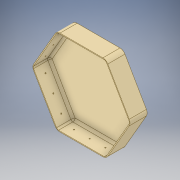
# Autodesk Inventor part: Base
Saved by Autodesk Inventor 2019 (Build 230136000, 136)
## iProperties
Created: 2021-07-14
Part Number: Base
Material: Generic
Document SubType Name: Modeling
Designer: Lix
Density: 1 g/cm^3
Appearance: Beige
Author: Lix
Autodesk Inventor part; units mm, degrees
ref_plane "YZ Plane" through (0, 0, 0) normal (1, 0, 0) x (0, 1, 0)
ref_plane "XZ Plane" through (0, 0, 0) normal (0, 1, 0) x (-1, 0, 0)
ref_plane "XY Plane" through (0, 0, 0) normal (0, 0, 1) x (1, 0, 0)
sketch "Sketch1" plane through (0, 0, 0) normal (0, 0, 1) x (1, 0, 0)
  line L0 (43.3013, -75) -> (-43.3013, -75)
  line L1 (-43.3013, -75) -> (-86.6025, 0)
  line L2 (-86.6025, 0) -> (-43.3013, 75)
  line L3 (-43.3013, 75) -> (43.3013, 75)
  line L4 (43.3013, 75) -> (86.6025, 0)
  line L5 (86.6025, 0) -> (43.3013, -75)
  point P0 (0, 0)
  point P1 (0, 0)
  dimension "d0" = 150
  constraints: 12 end point, 1 coincident, 1 horizontal, 13 other
  measures "d0" distance between parallel lines of L5 L2
extrude "Extrusion1" add sketch "Sketch1" along normal blind 30
shell "Shell1" thickness 1.5 removed faces 1 at (14.4338, -25, 30) ; own thickness 1 on faces at (14.4338, -25, 0)
sketch "Sketch2" plane through (-84.8705, 0, 30) normal (0.8660254, 0.5, 0) x (0, 0, -1)
  circle A0 centre (14.5, -69.8705) radius 1
  circle A1 centre (14.5, -15) radius 1
  line L0 (29, -84.8705) -> (0, -84.8705) projected
  line L1 (29, 0) -> (0, 0) projected
  circle A2 centre (14.5, -42.4352) radius 1
  line L2 (29, -84.8705) -> (29, 0) projected
  line L3 (29, 0) -> (0, 0) projected
  line L4 (0, -84.8705) -> (0, 0) projected
  line L5 (29, -84.8705) -> (0, -84.8705) projected
  line L6 (0, -84.8705) -> (0, 0) projected
  point P0 (30, -42.4352)
  point P1 (14.5, -84.8705)
  point P2 (0, -42.4352)
  dimension "d5" = 2
  dimension "d6" = 15
  dimension "d7" = 15
  constraints: 3 centre point, 3 vertical alignment, 2 equal radius, 2 midpoint, 1 horizontal alignment
  measures "d5" diameter of A0
  measures "d6" distance of A0.centre point (14.5, -84.87)
  measures "d7" distance from line of L1 A1.centre
ref_plane "Work Plane1" through (-21.6506, 37.5, 30) normal (0.8660254, 0.5, 0) x (0, 0, -1)
ref_plane "Work Plane2" through (-43.3013, 0, 0) normal (0, 1, 0) x (1, 0, 0)
ref_plane "Work Plane3" through (-21.6506, -37.5, 0) normal (-0.8660254, 0.5, 0) x (0, 0, 1)
extrude "Extrusion2" cut sketch "Sketch2" against normal blind 1 contours A0 | A1 | A2
mirror "Mirror1" about plane through (-21.6506, 37.5, 30) normal (0.8660254, 0.5, 0) of "Extrusion2"
mirror "Mirror2" about plane through (-43.3013, 0, 0) normal (0, 1, 0) of "Extrusion2"
mirror "Mirror3" about plane through (-21.6506, -37.5, 0) normal (-0.8660254, 0.5, 0) of "Extrusion2", "Mirror2"
mirror "Mirror4" about plane through (-43.3013, 0, 0) normal (0, 1, 0) of "Extrusion2", "Mirror2", "Mirror3"
fillet "Fillet1" radius 4 12 edges at (0, -73.5, 1) (-63.6529, -36.75, 1) (63.6529, -36.75, 1) (63.6529, 36.75, 1) (0, 73.5, 1) (-63.6529, 36.75, 1) (-84.8705, 0, 15.5) (-42.4352, 73.5, 15.5) (42.4352, 73.5, 15.5) (84.8705, 0, 15.5) (42.4352, -73.5, 15.5) (-42.4352, -73.5, 15.5)
fillet "Fillet2" radius 10 6 edges at (86.6025, 0, 15) (43.3013, 75, 15) (-43.3013, 75, 15) (43.3013, -75, 15) (-86.6025, 0, 15) (-43.3013, -75, 15)
equation "\"d7\" = d6"
body "Solid1"
